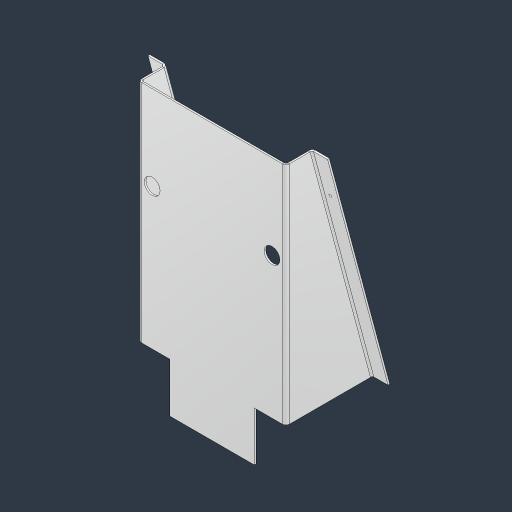
# Autodesk Inventor part: hopper_feeder
Saved by Autodesk Inventor 2024.3 (Build 283343000, 343)
## iProperties
Created: 2025-03-06
Part Number: hopper_feeder
Material: Aluminum 6061
Document SubType Name: Sheet Metal
Designer: Marcus Tannini
Density: 2.7 g/cm^3
Sheet Metal Rule: Default
Appearance: Aluminum - Flat
Mass: 1839.97 g
Surface Area: 4540.66 cm^2
Volume: 681.469 cm^3
Author: Marcus Tannini
Autodesk Inventor part; units mm, degrees
ref_plane "YZ Plane" through (0, 0, 0) normal (1, 0, 0) x (0, 1, 0)
ref_plane "XZ Plane" through (0, 0, 0) normal (0, 1, 0) x (-1, 0, 0)
ref_plane "XY Plane" through (0, 0, 0) normal (0, 0, 1) x (1, 0, 0)
sketch "Sketch1" plane through (0, 0, 0) normal (0, 0, 1) x (1, 0, 0)
  line L0 (127, -177.8) -> (-127, -177.8)
  line L1 (-127, -177.8) -> (-127, 177.8)
  line L2 (-127, 177.8) -> (127, 177.8)
  line L3 (127, 177.8) -> (127, -177.8)
  line L4 (127, -177.8) -> (-127, 177.8) construction
  line L5 (-127, -177.8) -> (127, 177.8) construction
  line L6 (76.2, -177.8) -> (-76.2, -177.8)
  line L7 (-76.2, -177.8) -> (-76.2, -266.7)
  line L8 (-76.2, -266.7) -> (76.2, -266.7)
  line L9 (76.2, -266.7) -> (76.2, -177.8)
  line L10 (127, 177.8) -> (-127, 177.8)
  line L11 (-127, 177.8) -> (-127, 228.6)
  line L12 (-127, 228.6) -> (127, 228.6)
  line L13 (127, 228.6) -> (127, 177.8)
  point P0 (0, 0)
  point P1 (0, -266.7)
  point P2 (0, -177.8)
  dimension "d0" = 254
  dimension "d1" = 355.6
  dimension "d47" = 152.4
  dimension "d48" = 88.9
  dimension "d49" = 50.8
  measures "d0" distance of L1.end L2.end
  measures "d1" distance of L0.end L1.end
  measures "d47" distance of L7.end L8.end
  measures "d48" distance of L8.end L6.start
  measures "d49" distance of L1.end L11.end
extrude "Plate1" add sketch "Sketch1" along normal blind 3.048
sketch "Sketch2" plane through (0, 0, 3.048) normal (0, 0, 1) x (1, 0, 0)
  line L0 (0, 0) -> (0, 25.4) construction
  point P0 (-107.95, 76.2)
  point P1 (107.95, 76.2)
  dimension "d3" = 25.4
  dimension "d4" = 107.95
  dimension "d5" = 76.2
  constraints: 2 end point, 1 symmetric about line, 1 vertical
  measures "d3" distance of L0.start L0.end
  measures "d4" horizontal distance of point (-107.95, 76.2) L0.start
  measures "d5" vertical distance of point (-107.95, 76.2) L0.start
hole "Hole1" at (-107.95, 76.2, 3.048) at (107.95, 76.2, 3.048) direction (0, 0, -1) diameter 28.575 end through all
sketch "Sketch3" plane through (-130.048, 228.6, -3.048) normal (-1, 0, 0) x (0, -1, 0)
  line L0 (406.4, 0) -> (0, 0)
  line L1 (0, 0) -> (0, -146.304)
  line L2 (0, -146.304) -> (406.4, -146.304)
  line L3 (406.4, -146.304) -> (406.4, 0)
  constraints: 6 end point, 1 horizontal, 1 perpendicular, 1 vertical
edge flange "Flange1" height 152.4 angle 90 thickness 3.048 bend radius 3.048 thickness toward (-1, 0, 0) relief tear relief width 3.048 relief depth 1.524 corner gap 3.048 corner form 0 edges at (-127, 25.4, 0) (127, 25.4, 0) wall of the first edge with corners at (-130.048, -177.8, -3.048) (-130.048, 228.6, -3.048) (-130.048, 228.6, -149.352) (-130.048, -177.8, -149.352)
bend "Bend1"
corner "Corner1"
sketch "Sketch4" plane through (133.096, -177.8, -149.352) normal (1, 0, 0) x (0, 0, -1)
  line L0 (0, 406.4) -> (0, 0) projected
  line L1 (0, 0) -> (-108.8946, 406.4)
  line L2 (0, 0) -> (420.7362, 0) construction
  line L3 (-146.304, 406.4) -> (0, 406.4) projected
  point P0 (-149.352, 177.8)
  dimension "d25" = 105
  constraints: 4 end point, 1 equal length, 1 horizontal, 1 point on line
  measures "d25" angle of L2 L1
extrude "Cut1" cut sketch "Sketch4" against normal through all
sketch "Sketch5" plane through (136.144, 229.3889, -43.4016) normal (0, 0.258819, -0.9659258) x (-1, 0, 0)
  line L0 (0, -420.7362) -> (0, 0)
  line L1 (0, 0) -> (-25.654, 0)
  line L2 (-25.654, 0) -> (-25.654, -420.7362)
  line L3 (-25.654, -420.7362) -> (0, -420.7362)
  constraints: 6 end point, 1 horizontal, 1 perpendicular, 1 vertical
edge flange "Flange2" height 31.75 angle 90 thickness 3.048 bend radius 3.048 thickness toward (0, 0.258819, -0.9659258) relief tear relief width 3.048 relief depth 1.524 corner gap 3.048 corner form 0 edges at (133.096, 25.4, -94.9047) (-133.096, 25.4, -94.9047) wall of the first edge with corners at (136.144, -177.0111, -152.2961) (136.144, 229.3889, -43.4016) (161.798, 229.3889, -43.4016) (161.798, -177.0111, -152.2961)
bend "Bend2"
corner "Corner2"
sketch "Sketch6" plane through (-161.798, 229.3889, -43.4016) normal (0, -0.258819, 0.9659258) x (1, 0, 0)
  line L0 (161.798, 14.783) -> (161.798, -196.5453) construction
  line L1 (14.9543, -76.2) -> (308.6418, -76.2)
  line L2 (0, 0) -> (25.654, 0) construction
  line L3 (34.798, 11.26) -> (288.798, 11.26) construction
  point P0 (161.798, -210.3395)
  point P1 (161.798, -76.2)
  point P2 (161.798, 11.26)
  dimension "d38" = 293.6875
  dimension "d50" = 76.2
  constraints: 4 end point, 2 midpoint, 2 vertical alignment, 1 parallel, 1 vertical
  measures "d38" distance of L1.start L1.end
  measures "d50" distance from line of L1.start L2
hole "Hole2" at (-146.8438, 155.7853, -63.1236) at (146.8437, 155.7853, -63.1236) direction (0, 0.258819, -0.9659258) diameter 5.1054 end through all clearance for "Flat Head Machine Screw (82)" size "#10" standard "Ansi Unified Screw Threads"
equation "\"d12\" = Thickness"
equation "\"d26\" = Thickness"
equation "\"d2\" = Thickness"
equation "\"d14\" = BendReliefWidth"
equation "\"d15\" = BendReliefDepth"
equation "\"d16\" = MinimumRemnant"
equation "\"d17\" = TransitionRadius"
equation "\"d20\" = BendRadius"
equation "\"d21\" = CornerReliefSize"
equation "\"d22\" = GapSize"
equation "\"d23\" = JacobiRadiusSize"
equation "\"d28\" = BendReliefWidth"
equation "\"d29\" = BendReliefDepth"
equation "\"d30\" = MinimumRemnant"
equation "\"d31\" = TransitionRadius"
equation "\"d34\" = BendRadius"
equation "\"d35\" = CornerReliefSize"
equation "\"d36\" = GapSize"
equation "\"d37\" = JacobiRadiusSize"
equation "\"BendRadius\" = Thickness"
equation "\"BendReliefWidth\" = Thickness"
equation "\"BendReliefDepth\" = 0.5 * Thickness"
equation "\"CornerReliefSize\" = 4 * Thickness"
equation "\"MinimumRemnant\" = 2 * Thickness"
equation "\"TransitionRadius\" = BendRadius"
equation "\"JacobiRadiusSize\" = BendRadius"
equation "\"GapSize\" = Thickness"
equation "\"Thickness\" = 3.048"
body "Solid1"
